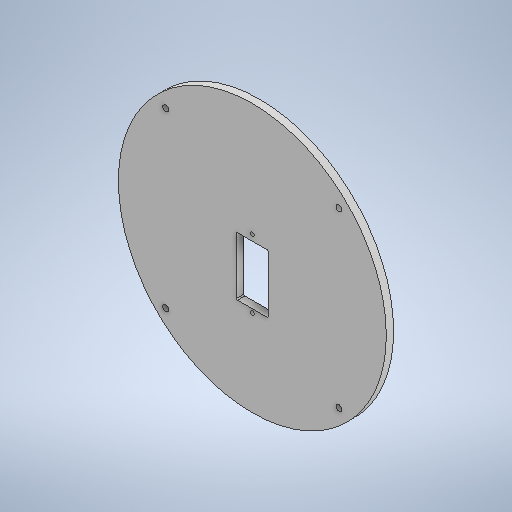
# Autodesk Inventor part: bottom-plate
Saved by Autodesk Inventor 2025 (Build 290162000, 162)
## iProperties
Created: 2024-05-28
Part Number: bottom-plate
Material: Generic
Document SubType Name: Modeling
Designer: hifzh
Density: 1 g/cm^3
Appearance: Default
Author: hifzh
Autodesk Inventor part; units mm, degrees
sketch "Sketch1" plane through (0, 0, 0) normal (0, 0, 1) x (1, 0, 0)
  circle A0 centre (0, 0) radius 55
  dimension "d0" = 110
  constraints: 1 centre point, 1 coincident
  measures "d0" diameter of A0
extrude "Extrusion1" add sketch "Sketch1" along normal blind 3
ref_plane "Work Plane1" through (0, 0, 4) normal (0, 0, 1) x (1, 0, 0)
sketch "Sketch2" plane through (0, 0, 4) normal (0, 0, 1) x (1, 0, 0)
  line L0 (-6.5, 6) -> (6.5, 6)
  line L1 (6.5, 6) -> (6.5, -18)
  line L2 (-6.5, -18) -> (-6.5, 6)
  circle A0 centre (-35.532, 35.532) radius 1.5
  circle A1 centre (-35.532, -35.532) radius 1.5
  circle A2 centre (35.532, -35.532) radius 1.5
  circle A3 centre (35.532, 35.532) radius 1.5
  line L3 (-6.5, -18) -> (6.5, -18)
  circle A4 centre (0, 8.5) radius 1
  circle A5 centre (0, -19.528) radius 1.9565
  point P0 (0, 0)
  point P1 (0, 6)
  point P2 (0, -13.848)
  dimension "d4" = 13
  dimension "d7" = 3
  dimension "d8" = 3
  dimension "d9" = 3
  dimension "d10" = 3
  dimension "d15" = 35.532
  dimension "d16" = 35.532
  dimension "d17" = 35.532
  dimension "d18" = 35.532
  dimension "d19" = 35.532
  dimension "d20" = 35.532
  dimension "d21" = 35.532
  dimension "d22" = 35.532
  dimension "d138" = 6
  dimension "d139" = 24
  dimension "d140" = 2
  dimension "d141" = 2.5
  dimension "d142" = 1.528
  constraints: 8 end point, 6 centre point, 2 horizontal, 1 midpoint, 1 parallel, 1 perpendicular, 1 vertical alignment
  measures "d4" distance of L0.start L0.end
  measures "d7" diameter of A0
  measures "d8" diameter of A1
  measures "d9" diameter of A2
  measures "d10" diameter of A3
  measures "d15" horizontal distance of point (0, 0) A0.centre
  measures "d16" horizontal distance of point (0, 0) A0.centre
  measures "d17" horizontal distance of point (0, 0) A3.centre
  measures "d18" horizontal distance of point (0, 0) A3.centre
  measures "d19" horizontal distance of point (0, 0) A2.centre
  measures "d20" horizontal distance of point (0, 0) A2.centre
  measures "d21" horizontal distance of point (0, 0) A1.centre
  measures "d22" horizontal distance of point (0, 0) A1.centre
  measures "d138" distance from line of point (0, 0) L0
  measures "d139" distance of L2.start L0.start
  measures "d140" diameter of A4
  measures "d141" distance of point (0, 6) A4.centre
  measures "d142" distance from line of L3 A5.centre
extrude "Extrusion2" cut sketch "Sketch2" against normal blind 4 contours L0 L1 L3 A5 L2 | A5 L3 picked at (0, -17.8572)
ref_plane "Work Plane2" through (0, 0, 3) normal (0, 0, 1) x (1, 0, 0)
sketch "Sketch3" plane through (0, 0, 3) normal (0, 0, 1) x (1, 0, 0)
  circle A0 centre (-35.577, 35.5342) radius 2.5
  circle A1 centre (-35.5225, -35.5931) radius 2.5
  circle A2 centre (35.5095, -35.5931) radius 2.5
  circle A3 centre (35.5095, 35.4262) radius 2.5
  point P0 (0, 0)
  constraints: 4 centre point
ref_plane "Work Plane3" through (0, 0, -1) normal (0, 0, 1) x (1, 0, 0)
ref_plane "Work Plane4" through (0, 0, 0) normal (0, 0, -1) x (-1, 0, 0)
sketch "Sketch5" plane through (0, 0, 0) normal (0, 0, -1) x (-1, 0, 0)
  line L0 (-9.906, 9.652) -> (9.906, 9.652)
  line L1 (9.906, 9.652) -> (9.906, -30.226)
  line L2 (9.906, -30.226) -> (-9.906, -30.226)
  line L3 (-9.906, -30.226) -> (-9.906, 9.652)
  circle A0 centre (-35.532, 35.532) radius 1.5
  circle A1 centre (-35.532, -35.532) radius 1.5
  circle A2 centre (35.532, -35.532) radius 1.5
  circle A3 centre (35.532, 35.532) radius 1.5
  circle A4 centre (-5.08, 13.462) radius 1
  circle A5 centre (5.08, 13.462) radius 1
  circle A6 centre (-5.08, -34.036) radius 1
  circle A7 centre (5.08, -34.036) radius 1
  point P0 (0, 0)
  point P1 (0, 0)
  point P2 (0, 9.652)
  point P3 (0, -30.226)
  dimension "d53" = 19.812
  dimension "d54" = 39.878
  dimension "d55" = 9.652
  dimension "d56" = 3
  dimension "d57" = 3
  dimension "d58" = 3
  dimension "d59" = 3
  dimension "d60" = 2
  dimension "d61" = 2
  dimension "d62" = 2
  dimension "d63" = 2
  dimension "d64" = 35.532
  dimension "d65" = 35.532
  dimension "d66" = 35.532
  dimension "d67" = 35.532
  dimension "d68" = 35.532
  dimension "d69" = 35.532
  dimension "d70" = 35.532
  dimension "d71" = 35.532
  dimension "d72" = 10.16
  dimension "d73" = 10.16
  dimension "d74" = 3.81
  dimension "d75" = 3.81
  dimension "d76" = 3.81
  dimension "d77" = 3.81
  dimension "d78" = 30.226
  dimension "d79" = 5.08
  dimension "d80" = 5.08
  dimension "d81" = 5.08
  dimension "d82" = 5.08
  constraints: 8 centre point, 8 end point, 2 midpoint, 2 parallel, 1 horizontal, 1 perpendicular, 1 vertical alignment
  measures "d53" distance of L0.start L0.end
  measures "d54" distance of L0.end L1.end
  measures "d55" distance from line of point (0, 0) L0
  measures "d56" diameter of A0
  measures "d57" diameter of A1
  measures "d58" diameter of A2
  measures "d59" diameter of A3
  measures "d60" diameter of A4
  measures "d61" diameter of A5
  measures "d62" diameter of A6
  measures "d63" diameter of A7
  measures "d64" horizontal distance of point (0, 0) A0.centre
  measures "d65" horizontal distance of point (0, 0) A0.centre
  measures "d66" horizontal distance of point (0, 0) A3.centre
  measures "d67" horizontal distance of point (0, 0) A3.centre
  measures "d68" horizontal distance of point (0, 0) A2.centre
  measures "d69" horizontal distance of point (0, 0) A2.centre
  measures "d70" horizontal distance of point (0, 0) A1.centre
  measures "d71" horizontal distance of point (0, 0) A1.centre
  measures "d72" distance of A5.centre A4.centre
  measures "d73" distance of A7.centre A6.centre
  measures "d74" distance from line of L0 A4.centre
  measures "d75" distance from line of L0 A5.centre
  measures "d76" distance from line of L2 A6.centre
  measures "d77" distance from line of L2 A7.centre
  measures "d78" distance of point (0, -30.226) point (0, 0)
  measures "d79" horizontal distance of point (0, 0) A5.centre
  measures "d80" horizontal distance of point (0, 0) A4.centre
  measures "d81" horizontal distance of point (0, 0) A7.centre
  measures "d82" horizontal distance of point (0, 0) A6.centre
hole "Hole1" at (35.532, 35.532, 0) at (-35.532, 35.532, 0) at (35.532, -35.532, 0) at (-35.532, -35.532, 0) direction (0, 0, 1) diameter 2.459 depth 4 tip angle 118 thread size "M3x0.5" class "6H" standard "ANSI Metric M Profile"
ref_plane "Work Plane5" through (0, 0, 0) normal (0, 0, -1) x (-1, 0, 0)
fillet "Fillet1" radius 0.4125 4 edges at (6.5, -18, 1.5) (-6.5, -18, 1.5) (6.5, 6, 1.5) (-6.5, 6, 1.5)
ref_plane "Work Plane6" through (0, 0, 0) normal (0, 0, -1) x (-1, 0, 0)
ref_plane "Work Plane7" through (0, 0, 3) normal (0, 0, 1) x (1, 0, 0)
sketch "Sketch8" plane through (0, 0, 3) normal (0, 0, 1) x (1, 0, 0)
  circle A0 centre (0, -19.528) radius 1
  circle A1 centre (0, 8.5) radius 1
  line L0 (6.0875, -18) -> (-6.0875, -18) projected
  line L1 (-6.0875, 6) -> (6.0875, 6) projected
  point P0 (0, 0)
  point P1 (0, -18)
  point P2 (0, -18)
  dimension "d144" = 2
  dimension "d145" = 2
  dimension "d146" = 1.528
  dimension "d147" = 2.5
  constraints: 2 centre point, 2 midpoint, 2 vertical alignment
  measures "d144" diameter of A0
  measures "d145" diameter of A1
  measures "d146" distance of point (0, -18) A0.centre
  measures "d147" distance from line of L1 A1.centre
hole "Hole3" at (0, 8.5, 3) at (0, -19.528, 3) direction (0, 0, -1) diameter 1.567 depth 6.3 tip angle 118 thread size "M2x0.4" class "6H" standard "ANSI Metric M Profile"
body "Solid1"
